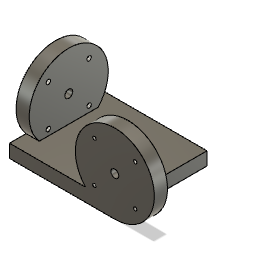
Link3 (Autodesk Fusion 360 design; units mm, degrees)
Autodesk Fusion 360 part; units mm, degrees
note: some values were not read from the file. Set by a fixed rule: which sketch regions a step uses.
sketch "Sketch1" plane through (0, 0, 0) normal (0, 0, 1) x (1, 0, 0)
  circle A0 centre (0, 0) radius 30
  dimension "d1" = 60
  constraint coincident A0.centre origin
  measures "d1" diameter of A0
extrude "Extrude1" add sketch "Sketch1" along normal blind 10
sketch "Sketch2" plane through (0, 0, 10) normal (0, 0, 1) x (1, 0, 0)
  circle A0 centre (0, 0) radius 30
  line L0 (0, -30) -> (-80, -30)
  line L1 (-80, -30) -> (-80, -20)
  line L2 (-80, -20) -> (0, -20)
  line L3 (0, -20) -> (0, -30)
  dimension "d4" = 80
  dimension "d5" = 10
  constraint horizontal L0
  constraint vertical L1
  constraint horizontal L2
  constraint vertical L3
  constraint coincident A0 L0.start
  constraint vertical A0.centre L0.start
  measures "d4" distance of L0.start L0.end
  measures "d5" distance of L0.start L2.end
extrude "Extrude2" add sketch "Sketch2" against normal blind 70 contours A0 L0 L1 L2 | A0 L2 L3 picked at (-1.3972, -26.5686)
sketch "Sketch3" plane through (-80, 0, 0) normal (-1, 0, 0) x (0, 0, 1)
  line L0 (10, -30) -> (10, -20)
  line L1 (10, -20) -> (-60, -20)
  line L2 (-60, -20) -> (-60, -30)
  line L3 (-60, -30) -> (10, -30)
  circle A0 centre (-25, 0) radius 30
  line L4 (-25, -30) -> (-25, 0) construction
  dimension "d8" = 60
  constraint horizontal origin A0.centre
  constraint midpoint L3 L4.start
  constraint coincident A0.centre L4.end
  constraint vertical L4
  measures "d8" diameter of A0
extrude "Extrude3" add sketch "Sketch3" against normal blind 10 contours L1 A0 picked at (-32.7403, 15.1228)
sketch "Sketch4" plane through (0, 0, 0) normal (0, 0, -1) x (-1, 0, 0)
  line L0 (0, -30) -> (0, -20)
  line L1 (0, -20) -> (22.3607, -20)
  arc A0 (22.3607, -20) -> (0, -30) centre (0, 0) ccw
  line L2 (15.5, -15.5) -> (-15.5, -15.5)
  line L3 (-15.5, -15.5) -> (-15.5, 15.5)
  line L4 (-15.5, 15.5) -> (15.5, 15.5)
  line L5 (15.5, 15.5) -> (15.5, -15.5)
  line L6 (15.5, -15.5) -> (-15.5, 15.5) construction
  line L7 (-15.5, -15.5) -> (15.5, 15.5) construction
  dimension "d11" = 31
  dimension "d12" = 31
  constraint horizontal L2
  constraint perpendicular L2 L3
  constraint parallel L2 L4
  constraint parallel L3 L5
  constraint coincident L6 A0.centre
  constraint coincident L7 A0.centre
  constraint coincident A0.centre origin
  measures "d11" distance of L3.end L4.end
  measures "d12" distance of L2.end L3.end
hole "Hole1" at (-15.5, 15.5, 0) at (15.5, 15.5, 0) at (15.5, -15.5, 0) at (-15.5, -15.5, 0) direction (0, 0, 1) diameter 2.529 depth 10 tip angle 118
thread "Thread1" "ISO Metric profile 3.0 M3x0.5 6H"
hole "Hole2" at (0, 0, 0) direction (0, 0, 1) diameter 6 depth 10 tip angle 118
sketch "Sketch5" plane through (-80, 0, 0) normal (-1, 0, 0) x (0, 0, 1)
  line L0 (10, -30) -> (10, -20)
  line L1 (10, -20) -> (-2.6393, -20)
  arc A0 (-2.6393, -20) -> (-47.3607, -20) centre (-25, 0) ccw
  line L2 (-47.3607, -20) -> (-60, -20)
  line L3 (-60, -20) -> (-60, -30)
  line L4 (-60, -30) -> (10, -30)
  line L5 (-40.5, 15.5) -> (-9.5, 15.5)
  line L6 (-9.5, 15.5) -> (-9.5, -15.5)
  line L7 (-9.5, -15.5) -> (-40.5, -15.5)
  line L8 (-40.5, -15.5) -> (-40.5, 15.5)
  line L9 (-40.5, 15.5) -> (-9.5, -15.5) construction
  line L10 (-9.5, 15.5) -> (-40.5, -15.5) construction
  point P0 (-25, 0)
  dimension "d19" = 31
  dimension "d20" = 31
  constraint horizontal L5
  constraint perpendicular L5 L6
  constraint parallel L5 L7
  constraint parallel L6 L8
  constraint coincident L9 P0
  constraint coincident L10 P0
  constraint coincident P0 A0.centre
  measures "d19" distance of L6.end L7.end
  measures "d20" distance of L5.end L6.end
hole "Hole3" at (-80, 15.5, -40.5) at (-80, 15.5, -9.5) at (-80, -15.5, -40.5) at (-80, -15.5, -9.5) direction (1, 0, 0) diameter 3.332 depth 40 tip angle 118
thread "Thread2" "ISO Metric profile 4.0 M4x0.7 6H"
hole "Hole4" at (-80, 0, -25) direction (1, 0, 0) diameter 6 depth 40 tip angle 118
